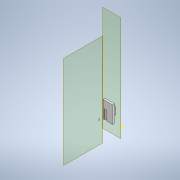
# Autodesk Inventor part: switch_b
Saved by Autodesk Inventor 2020 (Build 240168000, 168)
## iProperties
Created: 2020-03-15
Part Number: switch_b
Material: Generic
Document SubType Name: Modeling
Designer: erwin
Density: 1 g/cm^3
Appearance: Default
Author: erwin
Autodesk Inventor part; units mm, degrees
ref_plane "YZ Plane" through (0, 0, 0) normal (1, 0, 0) x (0, 1, 0)
ref_plane "XZ Plane" through (0, 0, 0) normal (0, 1, 0) x (-1, 0, 0)
ref_plane "XY Plane" through (0, 0, 0) normal (0, 0, 1) x (1, 0, 0)
ref_plane "Work Plane1" through (0, 0, -1.5) normal (0, 0, -1) x (-1, 0, 0)
sketch "Sketch1" plane through (0, 0, -1.5) normal (0, 0, -1) x (-1, 0, 0)
  line L0 (11.5, -60) -> (11.5, -65) projected
  arc A0 (9.3, -67.4819) -> (11.5, -65) centre (9, -65) ccw projected
  arc A1 (11.5, -60) -> (9.3, -57.5181) centre (9, -60) ccw projected
  line L1 (15, -75) -> (9.3, -75) projected
  line L2 (15, -5) -> (15, -75) projected
  line L3 (9.3, -5) -> (15, -5) projected
  line L4 (6.75, -60) -> (6.75, -65)
  arc A2 (6.75, -65) -> (11.25, -65) centre (9, -65) ccw
  line L5 (11.25, -65) -> (11.25, -60)
  arc A3 (11.25, -60) -> (6.75, -60) centre (9, -60) ccw
  line L6 (9, -65) -> (9, -61.5) construction
  line L7 (6.75, -65) -> (6.75, -61.5)
  line L8 (11.25, -61.5) -> (11.25, -65)
  arc A4 (6.75, -65) -> (11.25, -65) centre (9, -65) ccw
  arc A5 (11.25, -61.5) -> (6.75, -61.5) centre (9, -61.5) ccw
  line L9 (9.3, -57.5181) -> (9.3, -5) projected
  line L10 (9.3, -75) -> (9.3, -67.4819) projected
  point P0 (0, 0)
  point P1 (9, -63.25)
  dimension "d0" = 0.25
  dimension "d1" = 3.5
  constraints: 12 end point, 8 point on circle, 4 centre point, 4 tangent, 1 midpoint, 1 parallel, 1 vertical, 2 other
  measures "d0" radial gap between concentric circles of A1 A3
  measures "d1" distance of L6.start L6.end
extrude "Extrusion1" add sketch "Sketch1" along normal blind 0.5 and the other way blind 1.5 contours A5 L5 A2 L4
sketch "Sketch2" plane through (0, 0, 0) normal (0, 0, 1) x (1, 0, 0)
  line L0 (-6.75, -65) -> (-6.75, -61.5) projected
  arc A0 (-6.75, -61.5) -> (-11.25, -61.5) centre (-9, -61.5) ccw projected
  line L1 (-11.25, -61.5) -> (-11.25, -65) projected
  arc A1 (-11.25, -65) -> (-6.75, -65) centre (-9, -65) ccw projected
  line L2 (-12.5, -69.5) -> (-5.5, -69.5)
  line L3 (-5.5, -69.5) -> (-5.5, -60.5)
  line L4 (-5.5, -60.5) -> (-12.5, -60.5)
  line L5 (-12.5, -60.5) -> (-12.5, -69.5)
  line L6 (-12.5, -69.5) -> (-5.5, -60.5) construction
  line L7 (-5.5, -69.5) -> (-12.5, -60.5) construction
  line L8 (-12.5, -57) -> (-5.5, -57)
  line L9 (-5.5, -57) -> (-5.5, -66)
  line L10 (-5.5, -66) -> (-12.5, -66)
  line L11 (-12.5, -66) -> (-12.5, -57)
  line L12 (-12.5, -57) -> (-5.5, -66) construction
  line L13 (-5.5, -57) -> (-12.5, -66) construction
  point P0 (0, 0)
  dimension "d6" = 7
  dimension "d7" = 7
  dimension "d9" = 9
  constraints: 24 end point, 4 midpoint, 4 parallel, 2 horizontal, 2 perpendicular
  measures "d6" distance of L4.end L3.end
  measures "d7" distance of L9.end L10.end
  measures "d9" distance of L2.end L3.end
extrude "Extrusion2" add sketch "Sketch2" along normal blind 1
ref_plane "Work Plane2" through (-10.6833, -67.2, 6.3) normal (-1, 0, 0) x (0, 0, 1)
sketch "Sketch3" plane through (-10.6833, -67.2, 6.3) normal (-1, 0, 0) x (0, 0, 1)
  line L0 (0.322, -0.2398) -> (-0.378, -0.2398) projected
  line L1 (-0.378, -1.4398) -> (-0.378, -0.2398) projected
  line L2 (-0.378, -1.4398) -> (0.322, -1.4398) projected
  line L3 (0.322, -1.4398) -> (0.322, -0.2398) projected
  line L4 (0.272, 0.6602) -> (-1.028, 0.6602)
  line L5 (-1.028, 0.6602) -> (-1.028, -2.3398)
  line L6 (-1.028, -2.3398) -> (0.272, -2.3398)
  line L7 (0.272, -2.3398) -> (0.272, 0.6602)
  line L8 (0.272, 0.6602) -> (-1.028, -2.3398) construction
  line L9 (-1.028, 0.6602) -> (0.272, -2.3398) construction
  line L10 (-1.028, -2.3398) -> (-5.3, -2.3398)
  line L11 (0.272, 0.6602) -> (-5.3, 3.95)
  line L12 (-5.3, -2.3) -> (-5.3, 10.2) projected
  line L13 (-5.3, 3.95) -> (-5.3, -2.3398)
  point P0 (-6.3, 67.2)
  point P1 (-0.378, -0.8398)
  point P2 (-5.3, -0.9)
  point P3 (0.272, -1.4398)
  point P4 (0.272, -0.2398)
  dimension "d12" = 1.3
  dimension "d13" = 3
  constraints: 18 end point, 4 midpoint, 2 horizontal, 2 parallel, 1 collinear, 1 perpendicular
  measures "d12" distance of L6.end L5.end
  measures "d13" distance of L5.end L4.end
extrude "Extrusion3" add sketch "Sketch3" along normal mid plane 2 contours L0 L1 L2 L7 L6 L5 L4 | L4 L5 L10 L13 L12 L11
sketch "Sketch4" plane through (-12.5, -69.5, 0) normal (0, -1, 0) x (1, 0, 0)
  point P0 (12.5, 0)
move faces "Move1" translate (0, 0, 0.5) faces at (-6.8944, -63.25, 1)
ref_plane "Work Plane3" through (-9.4833, -47.5, 19.3) normal (-1, 0, 0) x (0, 0, 1)
sketch "Sketch5" plane through (-11.6833, -69.5398, 6.572) normal (0, -1, 0) x (1, 0, 0)
  line L0 (2, 0) -> (0, 0) projected
  line L1 (0, -5.572) -> (0, 0) projected
  line L2 (2, -5.572) -> (0, -5.572) projected
  line L3 (2, 0) -> (2, -5.572) projected
  point P0 (11.6833, -6.572)
extrude "Extrusion4" cut sketch "Sketch5" against normal blind 7
body "Solid1"
